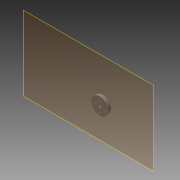
# Autodesk Inventor part: gearGuideDiscOutputStage1
Saved by Autodesk Inventor 2013 (Build 170138000, 138)
## iProperties
Created: 2014-07-01
Part Number: gearGuideDiscOutputStage1
Material: Generic
Document SubType Name: Modeling
Designer: Nano
Density: 1 g/cm^3
Author: Nano
Autodesk Inventor part; units mm, degrees
ref_plane "YZ Plane" through (0, 0, 0) normal (1, 0, 0) x (0, 1, 0)
ref_plane "XZ Plane" through (0, 0, 0) normal (0, 1, 0) x (-1, 0, 0)
ref_plane "XY Plane" through (0, 0, 0) normal (0, 0, 1) x (1, 0, 0)
ref_plane "Work Plane1" through (-7.9975, -173.6428, 0) normal (0, 0, 1) x (0.9989, -0.0477, 0)
sketch "Sketch1" plane through (-7.9975, -173.6428, 0) normal (0, 0, 1) x (0.9989, -0.0477, 0)
  circle A0 centre (24.871, 68.4391) radius 19.05 projected
  circle A1 centre (37.9927, 67.6226) radius 1.8542 projected
  circle A2 centre (25.6875, 81.5607) radius 1.8542 projected
  circle A3 centre (11.7494, 69.2555) radius 1.8542 projected
  circle A4 centre (24.0546, 55.3174) radius 1.8542 projected
  circle A5 centre (24.871, 68.4391) radius 3.175 projected
  point P0 (-0.2983, 173.8266)
extrude "Extrusion1" add sketch "Sketch1" against normal blind 6.35
body "Solid1"
